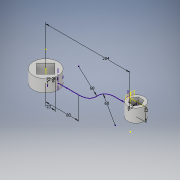
# Autodesk Inventor part: 練習三
Saved by Autodesk Inventor 2017 (Build 210142000, 142)
## iProperties
Part Number: 練習三
Material: 一般
Document SubType Name: Modeling
Designer: user
Density: 1 g/cm^3
Appearance: 預設
Author: user
Autodesk Inventor part; units mm, degrees
sketch "草圖1" plane through (0, 0, 0) normal (0, 1, 0) x (-1, 0, 0)
  circle A0 centre (0, 0) radius 30
  line L0 (0, 22.6274) -> (-22.6274, 0)
  line L1 (-22.6274, 0) -> (0, -22.6274)
  line L2 (0, -22.6274) -> (22.6274, 0)
  line L3 (22.6274, 0) -> (0, 22.6274)
  line L4 (17.214, 3.8392) -> (-17.214, -3.8392) construction
  line L5 (-19.542, 13.3062) -> (19.542, -13.3062) construction
  line L6 (11.3137, -11.3137) -> (-26.3636, 26.3636)
  line L7 (-11.3137, -11.3137) -> (19.159, 19.159)
  dimension "d0" = 60
  dimension "d1" = 32
  dimension "d2" = 32
  constraints: 16 end point, 6 midpoint, 3 parallel, 3 point on line, 2 perpendicular, 1 centre point, 1 coincident, 1 other
  measures "d0" diameter of A0
  measures "d1" distance between parallel lines of L2 L0
  measures "d2" distance between parallel lines of L1 L3
extrude "擠出1" add sketch "草圖1" along normal blind 30
ref_plane "工作平面1" through (0, 71, 0) normal (0, 1, 0) x (1, 0, 0)
sketch "草圖2" plane through (0, 71, 0) normal (0, 1, 0) x (1, 0, 0)
  circle A0 centre (220, 0) radius 20
  line L0 (233.8564, 0) -> (226.9282, -12)
  line L1 (226.9282, -12) -> (213.0718, -12)
  line L2 (213.0718, -12) -> (206.1436, 0)
  line L3 (206.1436, 0) -> (213.0718, 12)
  line L4 (213.0718, 12) -> (226.9282, 12)
  line L5 (226.9282, 12) -> (233.8564, 0)
  point P0 (0, 0)
  dimension "d14" = 220
  dimension "d15" = 40
  dimension "d16" = 0
  dimension "d17" = 24
  constraints: 12 end point, 1 centre point, 1 coincident, 1 horizontal, 13 other
  measures "d14" distance of A0.centre point (0, 0)
  measures "d15" diameter of A0
  measures "d16" vertical distance of A0.centre point (0, 0)
  measures "d17" distance between parallel lines of L4 L1
extrude "擠出2" add sketch "草圖2" against normal blind 32
sketch "草圖3" plane through (0, 0, 0) normal (0, 0, 1) x (1, 0, 0)
  line L0 (0, 0) -> (0, 30) projected
  line L1 (200, 71) -> (240, 71) projected
  line L2 (220, 71) -> (220, 39)
  arc A0 (169.4427, 55) -> (124.7214, 35) centre (169.4427, -5) ccw
  arc A1 (80, 15) -> (124.7214, 35) centre (80, 75) ccw
  line L3 (80, 15) -> (23, 15)
  line L4 (169.4427, 55) -> (204, 55)
  line L5 (204, 55) -> (204, 27.8796)
  point P0 (186.7214, 55)
  point P1 (220, 55)
  point P2 (51.5, 15)
  point P3 (0, 15)
  dimension "d39" = 32
  dimension "d40" = 60
  dimension "d41" = 60
  dimension "d58" = 23
  dimension "d59" = 80
  dimension "d60" = 204
  constraints: 8 end point, 5 midpoint, 4 point on circle, 3 tangent, 2 centre point, 2 horizontal, 2 horizontal alignment, 2 vertical
  measures "d39" distance of L2.start L2.end
  measures "d40" radius of A0
  measures "d41" radius of A1
  measures "d58" distance from line of L3.end L0
  measures "d59" distance from line of L0 L3.start
  measures "d60" distance from line of L4.end L0
sketch "草圖10" plane through (0, 0, 0) normal (0, 0, 1) x (1, 0, 0)
  line L0 (-30, 0) -> (30, 0) projected
  line L1 (30, 0) -> (30, 46.0087)
  line L2 (200, 39) -> (240, 39) projected
  line L3 (200, 39) -> (200, 88.733)
  point P0 (0, 0)
  constraints: 4 end point, 2 vertical
ref_plane "工作平面8" through (30, 0, 0) normal (1, 0, 0) x (0, 1, 0)
ref_plane "工作平面9" through (200, 39, 0) normal (-1, 0, 0) x (0, -1, 0)
sketch "草圖13" plane through (0, 30, 0) normal (0, 1, 0) x (1, 0, 0)
  point P0 (0, 0)
sketch "草圖14" plane through (220, 71, 0) normal (0, 1, 0) x (1, 0, 0)
  point P0 (-220, 0)
ref_plane "工作平面10" through (23, 15, 0) normal (-1, 0, 0) x (0, -1, 0)
sketch "草圖15" plane through (23, 15, 0) normal (-1, 0, 0) x (0, -1, 0)
  line L0 (15, 0) -> (-15, 0) projected
  ellipse E0 centre (0, 0) end of major axis (0, -19.261) minor radius 8
  dimension "d61" = 19.261
  dimension "d62" = 8
  constraints: 1 midpoint, 2 other
ref_plane "工作平面13" through (206.1436, 71, 0) normal (1, 0, 0) x (0, 1, 0)
sketch "草圖16" plane through (206.1436, 71, 0) normal (1, 0, 0) x (0, 1, 0)
  line L0 (-32, 0) -> (17.733, 0) projected
  ellipse E0 centre (-16, 0) end of major axis (-16, 12) minor radius 8
  point P0 (-71, 0)
  dimension "d63" = 8
  dimension "d64" = 12
  constraints: 1 coincident, 2 other
